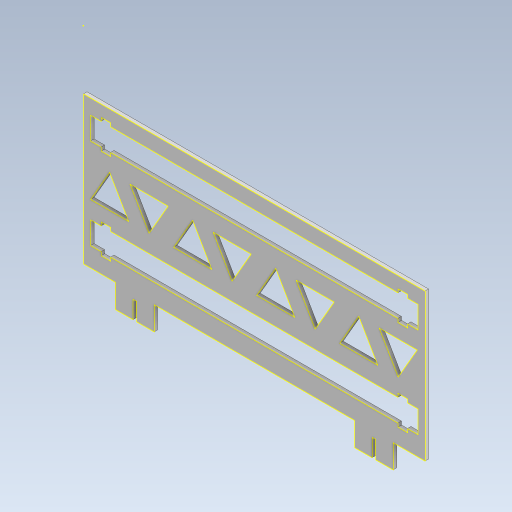
# Autodesk Inventor part: 零件5
Saved by Autodesk Inventor 2023 (Build 270158000, 158)
## iProperties
Created: 2023-05-12
Part Number: 零件5
Material: 一般
Document SubType Name: Modeling
Designer: Johnny Jou
Density: 1 g/cm^3
Appearance: 預設
Author: Johnny Jou
Autodesk Inventor part; units mm, degrees
ref_plane "YZ Plane" through (0, 0, 0) normal (1, 0, 0) x (0, 1, 0)
ref_plane "XZ Plane" through (0, 0, 0) normal (0, 1, 0) x (-1, 0, 0)
ref_plane "XY Plane" through (0, 0, 0) normal (0, 0, 1) x (1, 0, 0)
sketch "草圖1" plane through (0, 0, 0) normal (0, 0, 1) x (1, 0, 0)
  line L0 (0, 0) -> (290, 0)
  line L1 (290, 0) -> (290, -195)
  line L2 (290, -195) -> (0, -195)
  line L3 (0, -195) -> (0, 0)
  line L4 (15, -59.78) -> (23, -59.78)
  line L5 (23, -59.78) -> (23, -62.73)
  line L6 (23, -62.73) -> (15, -62.73)
  line L7 (15, -62.73) -> (15, -59.78)
  line L8 (15, -81.65) -> (23, -81.65)
  line L9 (23, -81.65) -> (23, -84.6)
  line L10 (23, -84.6) -> (15, -84.6)
  line L11 (15, -84.6) -> (15, -81.65)
  line L12 (15, -136.65) -> (23, -136.65)
  line L13 (23, -136.65) -> (23, -139.6)
  line L14 (23, -139.6) -> (15, -139.6)
  line L15 (15, -139.6) -> (15, -136.65)
  line L16 (15, -158.57) -> (23, -158.57)
  line L17 (23, -158.57) -> (23, -161.52)
  line L18 (23, -161.52) -> (15, -161.52)
  line L19 (15, -161.52) -> (15, -158.57)
  line L20 (275, -81.65) -> (275, -84.6)
  line L21 (275, -59.78) -> (275, -62.73)
  line L22 (267, -81.65) -> (275, -81.65)
  line L23 (275, -62.73) -> (267, -62.73)
  line L24 (267, -59.78) -> (275, -59.78)
  line L25 (275, -84.6) -> (267, -84.6)
  line L26 (267, -84.6) -> (267, -81.65)
  line L27 (267, -62.73) -> (267, -59.78)
  line L28 (267, -136.65) -> (275, -136.65)
  line L29 (275, -136.65) -> (275, -139.6)
  line L30 (267, -139.6) -> (267, -136.65)
  line L31 (275, -139.6) -> (267, -139.6)
  line L32 (267, -158.57) -> (275, -158.57)
  line L33 (275, -158.57) -> (275, -161.52)
  line L34 (275, -161.52) -> (267, -161.52)
  line L35 (267, -161.52) -> (267, -158.57)
  line L36 (0, -97.5) -> (290, -97.5) construction
  line L37 (19, -84.6) -> (19, -136.65) construction
  line L38 (145, 0) -> (145, -195) construction
  line L39 (23, -83.125) -> (267, -83.125) construction
  point P0 (15, -83.125)
  point P1 (15, -61.255)
  point P2 (15, -138.125)
  point P3 (15, -160.045)
  point P4 (267, -61.255)
  point P5 (267, -138.125)
  point P6 (267, -160.045)
  point P7 (145, -83.125)
  dimension "d0" = 2.95
  dimension "d1" = 8
  dimension "d3" = 55
  dimension "d5" = 195
  dimension "d6" = 290
  dimension "d9" = 252
  dimension "d16" = 12.9
  dimension "d36" = 18.92
  dimension "d37" = 18.97
  constraints: 80 end point, 12 midpoint, 11 point on line, 10 parallel, 6 horizontal, 6 perpendicular, 4 equal length, 36 other
  measures "d0" distance of L4.end L5.end
  measures "d1" distance of L4.start L4.end
  measures "d3" distance of point (15, -138.125) point (15, -83.125)
  measures "d5" distance of L0.end L1.end
  measures "d6" distance of L0.start L0.end
  measures "d9" distance of L5.end L21.end
  measures "d16" distance between parallel lines of L36 L10
  measures "d36" distance between parallel lines of L6 L8
  measures "d37" distance between parallel lines of L16 L14
extrude "擠出1" add sketch "草圖1" along normal blind 3
sketch "草圖3" plane through (0, 0, 3) normal (0, 0, 1) x (1, 0, 0)
  line L0 (290, 0) -> (0, 0) projected
  line L1 (0, 0) -> (290, 0)
  line L2 (290, 0) -> (290, -50)
  line L3 (290, -50) -> (0, -50)
  line L4 (0, -50) -> (0, 0)
  line L5 (290, -195) -> (290, 0) projected
  line L6 (42.05, -195) -> (45, -195)
  line L7 (45, -195) -> (45, -180)
  line L8 (45, -180) -> (42.05, -180)
  line L9 (42.05, -180) -> (42.05, -195)
  line L10 (0, -195) -> (290, -195) projected
  line L11 (245, -195) -> (247.95, -195)
  line L12 (247.95, -195) -> (247.95, -180)
  line L13 (247.95, -180) -> (245, -180)
  line L14 (245, -180) -> (245, -195)
  line L15 (45, -187.5) -> (245, -187.5)
  point P0 (145, -195)
  point P1 (145, -187.5)
  point P2 (247.95, -195)
  dimension "d17" = 50
  dimension "d18" = 200
  dimension "d19" = 2.95
  dimension "d20" = 2.95
  dimension "d22" = 15
  dimension "d23" = 0
  constraints: 26 end point, 6 parallel, 4 midpoint, 3 collinear, 3 horizontal, 3 perpendicular, 1 point on line
  measures "d17" distance of L1.end L2.end
  measures "d18" distance between parallel lines of L14 L7
  measures "d19" distance of L7.end L8.end
  measures "d20" distance of L12.end L13.end
  measures "d22" distance of L11.end L12.end
  measures "d23" horizontal distance of point (145, -195) point (145, -187.5)
extrude "擠出2" cut sketch "草圖3" against normal up to surface (3 mm away) contours L2 L3 L4 L0 | L9 L8 L7 L6 | L14 L13 L12 L10
sketch "草圖6" plane through (0, 0, 3) normal (0, 0, 1) x (1, 0, 0)
  line L0 (6, -139.6) -> (284, -139.6)
  line L1 (284, -139.6) -> (284, -158.57)
  line L2 (284, -158.57) -> (6, -158.57)
  line L3 (6, -158.57) -> (6, -139.6)
  line L4 (23, -139.6) -> (15, -139.6) projected
  line L5 (15, -158.57) -> (23, -158.57) projected
  line L6 (0, -50) -> (0, -195) projected
  line L7 (290, -195) -> (290, -50) projected
  line L8 (6, -81.65) -> (6, -62.73)
  line L9 (6, -62.73) -> (284, -62.73)
  line L10 (284, -62.73) -> (284, -81.65)
  line L11 (284, -81.65) -> (6, -81.65)
  line L12 (15, -81.65) -> (23, -81.65) projected
  line L13 (23, -62.73) -> (15, -62.73) projected
  line L14 (22.1369, -96.65) -> (38.2739, -124.6)
  line L15 (38.2739, -124.6) -> (6, -124.6)
  line L16 (6, -124.6) -> (22.1369, -96.65)
  line L17 (39.4574, -96.65) -> (71.7313, -96.65)
  line L18 (71.7313, -96.65) -> (55.5944, -124.6)
  line L19 (55.5944, -124.6) -> (39.4574, -96.65)
  line L20 (108.7739, -124.6) -> (76.5, -124.6)
  line L21 (76.5, -124.6) -> (92.6369, -96.65)
  line L22 (92.6369, -96.65) -> (108.7739, -124.6)
  line L23 (126.0944, -124.6) -> (109.9574, -96.65)
  line L24 (142.2313, -96.65) -> (126.0944, -124.6)
  line L25 (109.9574, -96.65) -> (142.2313, -96.65)
  line L26 (179.2739, -124.6) -> (147, -124.6)
  line L27 (147, -124.6) -> (163.1369, -96.65)
  line L28 (163.1369, -96.65) -> (179.2739, -124.6)
  line L29 (196.5944, -124.6) -> (180.4574, -96.65)
  line L30 (212.7313, -96.65) -> (196.5944, -124.6)
  line L31 (180.4574, -96.65) -> (212.7313, -96.65)
  line L32 (249.7739, -124.6) -> (217.5, -124.6)
  line L33 (217.5, -124.6) -> (233.6369, -96.65)
  line L34 (233.6369, -96.65) -> (249.7739, -124.6)
  line L35 (267.0944, -124.6) -> (250.9574, -96.65)
  line L36 (283.2313, -96.65) -> (267.0944, -124.6)
  line L37 (250.9574, -96.65) -> (283.2313, -96.65)
  line L38 (45, -195) -> (245, -195) projected
  line L39 (60, -195) -> (230, -195)
  line L40 (230, -195) -> (230, -175)
  line L41 (230, -175) -> (60, -175)
  line L42 (60, -175) -> (60, -195)
  line L43 (262.95, -195) -> (290, -195)
  line L44 (290, -195) -> (290, -175)
  line L45 (290, -175) -> (262.95, -175)
  line L46 (262.95, -175) -> (262.95, -195)
  line L47 (0, -195) -> (42.05, -195) projected
  line L48 (27.05, -195) -> (0, -195)
  line L49 (0, -195) -> (0, -175)
  line L50 (0, -175) -> (27.05, -175)
  line L51 (27.05, -175) -> (27.05, -195)
  line L52 (42.05, -195) -> (42.05, -180) projected
  line L53 (45, -180) -> (45, -195) projected
  line L54 (245, -195) -> (245, -180) projected
  line L55 (247.95, -180) -> (247.95, -195) projected
  point P0 (0, 0)
  point P1 (284, -149.085)
  point P2 (22.1369, -115.2833)
  point P3 (55.5944, -105.9667)
  point P4 (126.0944, -105.9667)
  point P5 (92.6369, -115.2833)
  point P6 (196.5944, -105.9667)
  point P7 (163.1369, -115.2833)
  point P8 (267.0944, -105.9667)
  point P9 (233.6369, -115.2833)
  point P10 (42.05, -187.5)
  dimension "d32" = 6
  dimension "d33" = 6
  dimension "d39" = 15
  dimension "d40" = 15
  dimension "d41" = 15
  dimension "d44" = 70.5
  dimension "d49" = 20
  dimension "d50" = 15
  dimension "d51" = 15
  dimension "d52" = 15
  dimension "d53" = 15
  constraints: 88 end point, 12 parallel, 8 collinear, 5 horizontal, 5 perpendicular, 5 point on line, 2 midpoint, 1 equal length, 1 horizontal alignment, 1 vertical, 1 vertical alignment, 56 other
  measures "d32" distance between parallel lines of L6 L3
  measures "d33" distance from line of L7 point (284, -149.085)
  measures "d39" distance between parallel lines of L19 L14
  measures "d40" distance between parallel lines of L11 L17
  measures "d41" distance between parallel lines of L4 L15
  measures "d44" distance of L14.end L20.start
  measures "d49" distance between parallel lines of L47 L50
  measures "d50" distance from line of point (42.05, -187.5) L51
  measures "d51" distance between parallel lines of L42 L53
  measures "d52" distance between parallel lines of L54 L40
  measures "d53" distance between parallel lines of L46 L55
extrude "擠出5" cut sketch "草圖6" against normal up to surface (3 mm away)
sketch "草圖8" plane through (0, 0, 3) normal (0, 0, 1) x (1, 0, 0)
  line L0 (275, -62.73) -> (284, -62.73) projected
  line L1 (284, -62.73) -> (284, -81.65) projected
  line L2 (284, -81.65) -> (275, -81.65) projected
  line L3 (275, -81.65) -> (275, -84.6) projected
  line L4 (275, -84.6) -> (267, -84.6) projected
  line L5 (267, -84.6) -> (267, -81.65) projected
  line L6 (267, -81.65) -> (23, -81.65) projected
  line L7 (23, -81.65) -> (23, -84.6) projected
  line L8 (23, -84.6) -> (15, -84.6) projected
  line L9 (15, -84.6) -> (15, -81.65) projected
  line L10 (15, -81.65) -> (6, -81.65) projected
  line L11 (6, -81.65) -> (6, -62.73) projected
  line L12 (6, -62.73) -> (15, -62.73) projected
  line L13 (15, -62.73) -> (15, -59.78) projected
  line L14 (15, -59.78) -> (23, -59.78) projected
  line L15 (23, -59.78) -> (23, -62.73) projected
  line L16 (23, -62.73) -> (267, -62.73) projected
  line L17 (267, -62.73) -> (267, -59.78) projected
  line L18 (267, -59.78) -> (275, -59.78) projected
  line L19 (275, -59.78) -> (275, -62.73) projected
  line L20 (15, -158.57) -> (6, -158.57) projected
  line L21 (6, -158.57) -> (6, -139.6) projected
  line L22 (6, -139.6) -> (15, -139.6) projected
  line L23 (15, -139.6) -> (15, -136.65) projected
  line L24 (15, -136.65) -> (23, -136.65) projected
  line L25 (23, -136.65) -> (23, -139.6) projected
  line L26 (23, -139.6) -> (267, -139.6) projected
  line L27 (267, -139.6) -> (267, -136.65) projected
  line L28 (267, -136.65) -> (275, -136.65) projected
  line L29 (275, -136.65) -> (275, -139.6) projected
  line L30 (275, -139.6) -> (284, -139.6) projected
  line L31 (284, -139.6) -> (284, -158.57) projected
  line L32 (284, -158.57) -> (275, -158.57) projected
  line L33 (275, -158.57) -> (275, -161.52) projected
  line L34 (275, -161.52) -> (267, -161.52) projected
  line L35 (267, -161.52) -> (267, -158.57) projected
  line L36 (267, -158.57) -> (23, -158.57) projected
  line L37 (23, -158.57) -> (23, -161.52) projected
  line L38 (23, -161.52) -> (15, -161.52) projected
  line L39 (15, -161.52) -> (15, -158.57) projected
  line L40 (55.5944, -124.6) -> (39.4574, -96.65) projected
  line L41 (39.4574, -96.65) -> (71.7313, -96.65) projected
  line L42 (71.7313, -96.65) -> (55.5944, -124.6) projected
  line L43 (212.7313, -96.65) -> (196.5944, -124.6) projected
  line L44 (196.5944, -124.6) -> (180.4574, -96.65) projected
  line L45 (180.4574, -96.65) -> (212.7313, -96.65) projected
  line L46 (109.9574, -96.65) -> (142.2313, -96.65) projected
  line L47 (142.2313, -96.65) -> (126.0944, -124.6) projected
  line L48 (126.0944, -124.6) -> (109.9574, -96.65) projected
  line L49 (250.9574, -96.65) -> (283.2313, -96.65) projected
  line L50 (283.2313, -96.65) -> (267.0944, -124.6) projected
  line L51 (267.0944, -124.6) -> (250.9574, -96.65) projected
  line L52 (92.6369, -96.65) -> (108.7739, -124.6) projected
  line L53 (108.7739, -124.6) -> (76.5, -124.6) projected
  line L54 (76.5, -124.6) -> (92.6369, -96.65) projected
  line L55 (147, -124.6) -> (163.1369, -96.65) projected
  line L56 (163.1369, -96.65) -> (179.2739, -124.6) projected
  line L57 (179.2739, -124.6) -> (147, -124.6) projected
  line L58 (38.2739, -124.6) -> (6, -124.6) projected
  line L59 (6, -124.6) -> (22.1369, -96.65) projected
  line L60 (22.1369, -96.65) -> (38.2739, -124.6) projected
  line L61 (217.5, -124.6) -> (233.6369, -96.65) projected
  line L62 (233.6369, -96.65) -> (249.7739, -124.6) projected
  line L63 (249.7739, -124.6) -> (217.5, -124.6) projected
  line L64 (262.95, -195) -> (262.95, -175) projected
  line L65 (262.95, -175) -> (290, -175) projected
  line L66 (290, -175) -> (290, -50) projected
  line L67 (290, -50) -> (0, -50) projected
  line L68 (0, -50) -> (0, -175) projected
  line L69 (0, -175) -> (27.05, -175) projected
  line L70 (27.05, -175) -> (27.05, -195) projected
  line L71 (27.05, -195) -> (42.05, -195) projected
  line L72 (42.05, -195) -> (42.05, -180) projected
  line L73 (42.05, -180) -> (45, -180) projected
  line L74 (45, -180) -> (45, -195) projected
  line L75 (45, -195) -> (60, -195) projected
  line L76 (60, -195) -> (60, -175) projected
  line L77 (60, -175) -> (230, -175) projected
  line L78 (230, -175) -> (230, -195) projected
  line L79 (230, -195) -> (245, -195) projected
  line L80 (245, -195) -> (245, -180) projected
  line L81 (245, -180) -> (247.95, -180) projected
  line L82 (247.95, -180) -> (247.95, -195) projected
  line L83 (247.95, -195) -> (262.95, -195) projected
  point P0 (0, 0)
